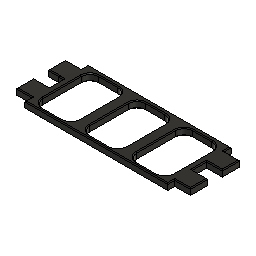
Ansamblu Final (Autodesk Fusion 360 archive; units mm, degrees)
design "Cadran Numere"
part number: 2026-05-27-02-16-51-186
Autodesk Fusion 360 part; units mm, degrees
(part 1 of 3)
sketch "Sketch1" plane through (0, 0, 0) normal (0, 0, 1) x (1, 0, 0)
  line L0 (40, 20) -> (128, 20)
  line L1 (40, 20) -> (40, 24)
  line L2 (40, 24) -> (34, 24)
  line L3 (34, 24) -> (34, 34)
  line L4 (34, 34) -> (40, 34)
  line L5 (40, 34) -> (40, 42.3)
  line L6 (40, 42.3) -> (34, 42.3)
  line L7 (34, 42.3) -> (34, 52.3)
  line L8 (34, 52.3) -> (40, 52.3)
  line L9 (40, 52.3) -> (40, 56.3)
  line L10 (40, 56.3) -> (128, 56.3)
  line L11 (128, 56.3) -> (128, 52.3)
  line L12 (128, 52.3) -> (134, 52.3)
  line L13 (134, 52.3) -> (134, 42.3)
  line L14 (134, 42.3) -> (128, 42.3)
  line L15 (128, 42.3) -> (128, 34)
  line L16 (128, 34) -> (134, 34)
  line L17 (134, 34) -> (134, 24)
  line L18 (134, 24) -> (128, 24)
  line L19 (128, 24) -> (128, 20)
  line L20 (51.5, 53.8) -> (62.5, 53.8)
  line L21 (67.5, 48.8) -> (67.5, 26.8)
  line L22 (62.5, 21.8) -> (51.5, 21.8)
  line L23 (46.5, 26.8) -> (46.5, 48.8)
  line L24 (78.5, 53.8) -> (89.5, 53.8)
  line L25 (94.5, 48.8) -> (94.5, 26.8)
  line L26 (89.5, 21.8) -> (78.5, 21.8)
  line L27 (73.5, 26.8) -> (73.5, 48.8)
  line L28 (105.5, 53.8) -> (116.5, 53.8)
  line L29 (121.5, 48.8) -> (121.5, 26.8)
  line L30 (116.5, 21.8) -> (105.5, 21.8)
  line L31 (100.5, 26.8) -> (100.5, 48.8)
  arc A0 (51.5, 53.8) -> (46.5, 48.8) centre (51.5, 48.8) ccw
  arc A1 (67.5, 48.8) -> (62.5, 53.8) centre (62.5, 48.8) ccw
  arc A2 (46.5, 26.8) -> (51.5, 21.8) centre (51.5, 26.8) ccw
  arc A3 (62.5, 21.8) -> (67.5, 26.8) centre (62.5, 26.8) ccw
  arc A4 (78.5, 53.8) -> (73.5, 48.8) centre (78.5, 48.8) ccw
  arc A5 (73.5, 26.8) -> (78.5, 21.8) centre (78.5, 26.8) ccw
  arc A6 (89.5, 21.8) -> (94.5, 26.8) centre (89.5, 26.8) ccw
  arc A7 (94.5, 48.8) -> (89.5, 53.8) centre (89.5, 48.8) ccw
  arc A8 (105.5, 53.8) -> (100.5, 48.8) centre (105.5, 48.8) ccw
  arc A9 (121.5, 48.8) -> (116.5, 53.8) centre (116.5, 48.8) ccw
  arc A10 (100.5, 26.8) -> (105.5, 21.8) centre (105.5, 26.8) ccw
  arc A11 (116.5, 21.8) -> (121.5, 26.8) centre (116.5, 26.8) ccw
  point P0 (46.5, 53.8)
  point P1 (67.5, 53.8)
  point P2 (46.5, 21.8)
  point P3 (73.5, 53.8)
  point P4 (94.5, 53.8)
  point P5 (73.5, 21.8)
  point P6 (100.5, 53.8)
  point P7 (121.5, 53.8)
  point P8 (100.5, 21.8)
  dimension "d1" = 88
  dimension "d2" = 4
  dimension "d3" = 6
  dimension "d4" = 10
  dimension "d5" = 6
  dimension "d6" = 8.3
  dimension "d7" = 6
  dimension "d8" = 10
  dimension "d9" = 6
  dimension "d10" = 4
  dimension "d11" = 88
  dimension "d12" = 4
  dimension "d13" = 6
  dimension "d14" = 10
  dimension "d15" = 6
  dimension "d16" = 8.3
  dimension "d17" = 6
  dimension "d18" = 10
  dimension "d21" = 21
  dimension "d22" = 32
  dimension "d23" = 6
  dimension "d24" = 21
  dimension "d25" = 32
  dimension "d26" = 6
  dimension "d27" = 21
  dimension "d28" = 32
  dimension "d29" = 5
  constraint horizontal L0
  constraint perpendicular L0 L1
  constraint perpendicular L1 L2
  constraint perpendicular L2 L3
  constraint perpendicular L3 L4
  constraint perpendicular L4 L5
  constraint perpendicular L5 L6
  constraint perpendicular L6 L7
  constraint perpendicular L7 L8
  constraint perpendicular L8 L9
  constraint perpendicular L9 L10
  constraint perpendicular L10 L11
  constraint perpendicular L11 L12
  constraint perpendicular L12 L13
  constraint perpendicular L13 L14
  constraint perpendicular L14 L15
  constraint perpendicular L15 L16
  constraint perpendicular L16 L17
  constraint perpendicular L17 L18
  constraint horizontal L20
  constraint vertical L21
  constraint horizontal L22
  constraint vertical L23
  constraint horizontal L24
  constraint vertical L25
  constraint horizontal L26
  constraint vertical L27
  constraint horizontal L28
  constraint vertical L29
  constraint horizontal L30
  constraint vertical L31
  constraint coincident P0 L20
  constraint coincident P0 L23
  constraint tangent L20 A0
  constraint tangent L23 A0
  constraint coincident P1 L20
  constraint coincident P1 L21
  constraint tangent L20 A1
  constraint tangent L21 A1
  constraint equal A0 A1
  constraint coincident P2 L23
  constraint coincident P2 L22
  constraint tangent L23 A2
  constraint tangent L22 A2
  constraint equal A0 A2
  constraint tangent L21 A3
  constraint tangent L22 A3
  constraint equal A0 A3
  constraint coincident P3 L24
  constraint coincident P3 L27
  constraint tangent L24 A4
  constraint tangent L27 A4
  constraint equal A0 A4
  constraint coincident P5 L27
  constraint coincident P5 L26
  constraint tangent L27 A5
  constraint tangent L26 A5
  constraint equal A0 A5
  constraint tangent L26 A6
  constraint tangent L25 A6
  constraint equal A0 A6
  constraint coincident P4 L25
  constraint coincident P4 L24
  constraint tangent L25 A7
  constraint tangent L24 A7
  constraint equal A0 A7
  constraint coincident P6 L28
  constraint coincident P6 L31
  constraint tangent L28 A8
  constraint tangent L31 A8
  constraint equal A0 A8
  constraint coincident P7 L28
  constraint coincident P7 L29
  constraint tangent L28 A9
  constraint tangent L29 A9
  constraint equal A0 A9
  constraint coincident P8 L31
  constraint coincident P8 L30
  constraint tangent L31 A10
  constraint tangent L30 A10
  constraint equal A0 A10
  constraint tangent L29 A11
  constraint tangent L30 A11
  constraint equal A0 A11
  measures "d1" distance of L0.start L0.end
  measures "d2" distance of L0.start L1.end
  measures "d3" distance of L1.end L2.end
  measures "d4" distance of L2.end L3.end
  measures "d5" distance of L3.end L4.end
  measures "d6" distance of L4.end L5.end
  measures "d7" distance of L5.end L6.end
  measures "d8" distance of L6.end L7.end
  measures "d9" distance of L7.end L8.end
  measures "d10" distance of L8.end L9.end
  measures "d11" distance of L9.end L10.end
  measures "d12" distance of L10.end L11.end
  measures "d13" distance of L11.end L12.end
  measures "d14" distance of L12.end L13.end
  measures "d15" distance of L13.end L14.end
  measures "d16" distance of L14.end L15.end
  measures "d17" distance of L15.end L16.end
  measures "d18" distance of L16.end L17.end
  measures "d21" distance of P0 P1
  measures "d22" distance of P0 P2
  measures "d23" distance of P1 P3
  measures "d24" distance of P3 P4
  measures "d25" distance of P3 P5
  measures "d26" distance of P4 P6
  measures "d27" distance of P6 P7
  measures "d28" distance of P6 P8
  measures "d29" radius of A0
extrude "Extrude1" add sketch "Sketch1" along normal blind 4
sketch "Sketch2" plane through (0, 0, 4) normal (0, 0, 1) x (-1, 0, 0)
  arc A0 (-100.5, -26.8) -> (-105.5, -21.8) centre (-105.5, -26.8) ccw
  line L0 (-100.5, -26.8) -> (-100.5, -48.8)
  arc A1 (-105.5, -53.8) -> (-100.5, -48.8) centre (-105.5, -48.8) ccw
  line L1 (-105.5, -53.8) -> (-116.5, -53.8)
  arc A2 (-121.5, -48.8) -> (-116.5, -53.8) centre (-116.5, -48.8) ccw
  line L2 (-121.5, -48.8) -> (-121.5, -26.8)
  arc A3 (-116.5, -21.8) -> (-121.5, -26.8) centre (-116.5, -26.8) ccw
  line L3 (-116.5, -21.8) -> (-105.5, -21.8)
  arc A4 (-89.5, -21.8) -> (-94.5, -26.8) centre (-89.5, -26.8) ccw
  line L4 (-89.5, -21.8) -> (-78.5, -21.8)
  arc A5 (-73.5, -26.8) -> (-78.5, -21.8) centre (-78.5, -26.8) ccw
  line L5 (-73.5, -26.8) -> (-73.5, -48.8)
  arc A6 (-78.5, -53.8) -> (-73.5, -48.8) centre (-78.5, -48.8) ccw
  line L6 (-78.5, -53.8) -> (-89.5, -53.8)
  arc A7 (-94.5, -48.8) -> (-89.5, -53.8) centre (-89.5, -48.8) ccw
  line L7 (-94.5, -48.8) -> (-94.5, -26.8)
  arc A8 (-46.5, -26.8) -> (-51.5, -21.8) centre (-51.5, -26.8) ccw
  line L8 (-46.5, -26.8) -> (-46.5, -48.8)
  arc A9 (-51.5, -53.8) -> (-46.5, -48.8) centre (-51.5, -48.8) ccw
  line L9 (-51.5, -53.8) -> (-62.5, -53.8)
  arc A10 (-67.5, -48.8) -> (-62.5, -53.8) centre (-62.5, -48.8) ccw
  line L10 (-67.5, -48.8) -> (-67.5, -26.8)
  arc A11 (-62.5, -21.8) -> (-67.5, -26.8) centre (-62.5, -26.8) ccw
  line L11 (-62.5, -21.8) -> (-51.5, -21.8)
  line L12 (-40, -20) -> (-128, -20)
  line L13 (-128, -20) -> (-128, -24)
  line L14 (-128, -24) -> (-134, -24)
  line L15 (-134, -24) -> (-134, -34)
  line L16 (-134, -34) -> (-128, -34)
  line L17 (-128, -34) -> (-128, -42.3)
  line L18 (-128, -42.3) -> (-134, -42.3)
  line L19 (-134, -42.3) -> (-134, -52.3)
  line L20 (-134, -52.3) -> (-128, -52.3)
  line L21 (-128, -52.3) -> (-128, -56.3)
  line L22 (-128, -56.3) -> (-40, -56.3)
  line L23 (-40, -56.3) -> (-40, -52.3)
  line L24 (-40, -52.3) -> (-34, -52.3)
  line L25 (-34, -52.3) -> (-34, -42.3)
  line L26 (-34, -42.3) -> (-40, -42.3)
  line L27 (-40, -42.3) -> (-40, -34)
  line L28 (-40, -34) -> (-34, -34)
  line L29 (-34, -34) -> (-34, -24)
  line L30 (-34, -24) -> (-40, -24)
  line L31 (-40, -24) -> (-40, -20)
  line L32 (-40, -56.3) -> (-43, -56.3)
  line L33 (-43, -56.3) -> (-43, -20)
  line L34 (-43, -20) -> (-40, -20)
  line L35 (-40, -20) -> (-40, -56.3)
  line L36 (-128, -56.3) -> (-125, -56.3)
  line L37 (-125, -56.3) -> (-125, -20)
  line L38 (-125, -20) -> (-128, -20)
  line L39 (-128, -20) -> (-128, -56.3)
  line L40 (-128, -52.3) -> (-125, -52.3)
  line L41 (-125, -52.3) -> (-125, -42.3)
  line L42 (-125, -42.3) -> (-128, -42.3)
  line L43 (-128, -42.3) -> (-128, -52.3)
  line L44 (-128, -34) -> (-125, -34)
  line L45 (-125, -34) -> (-125, -24)
  line L46 (-125, -24) -> (-128, -24)
  line L47 (-128, -24) -> (-128, -34)
  line L48 (-40, -52.3) -> (-43, -52.3)
  line L49 (-43, -52.3) -> (-43, -42)
  line L50 (-43, -42) -> (-40, -42)
  line L51 (-40, -42) -> (-40, -52.3)
  line L52 (-40, -34) -> (-43, -34)
  line L53 (-43, -34) -> (-43, -24)
  line L54 (-43, -24) -> (-40, -24)
  line L55 (-40, -24) -> (-40, -34)
  line L56 (-40, -42) -> (-43, -42)
  line L57 (-43, -42) -> (-43, -34)
  line L58 (-43, -34) -> (-40, -34)
  line L59 (-40, -34) -> (-40, -42)
  line L60 (-40, -56.3) -> (-43, -56.3)
  line L61 (-43, -56.3) -> (-43, -52.3)
  line L62 (-43, -52.3) -> (-40, -52.3)
  line L63 (-40, -52.3) -> (-40, -56.3)
  line L64 (-40, -24) -> (-43, -24)
  line L65 (-43, -24) -> (-43, -20)
  line L66 (-43, -20) -> (-40, -20)
  line L67 (-40, -20) -> (-40, -24)
  line L68 (-125, -56.3) -> (-128, -56.3)
  line L69 (-128, -56.3) -> (-128, -52.3)
  line L70 (-128, -52.3) -> (-125, -52.3)
  line L71 (-125, -52.3) -> (-125, -56.3)
  line L72 (-125, -42.3) -> (-128, -42.3)
  line L73 (-128, -42.3) -> (-128, -34)
  line L74 (-128, -34) -> (-125, -34)
  line L75 (-125, -34) -> (-125, -42.3)
  line L76 (-125, -24) -> (-128, -24)
  line L77 (-128, -24) -> (-128, -20)
  line L78 (-128, -20) -> (-125, -20)
  line L79 (-125, -20) -> (-125, -24)
  constraint horizontal L32
  constraint vertical L33
  constraint horizontal L34
  constraint vertical L35
  constraint coincident L12 L33.end
  constraint coincident L22.end L23.start
  constraint horizontal L36
  constraint vertical L37
  constraint horizontal L38
  constraint vertical L39
  constraint coincident L12 L37.end
  constraint coincident L21.end L22.start
  constraint horizontal L40
  constraint vertical L41
  constraint horizontal L42
  constraint vertical L43
  constraint coincident L37 L41.end
  constraint coincident L20.end L21.start
  constraint horizontal L44
  constraint vertical L45
  constraint horizontal L46
  constraint vertical L47
  constraint coincident L37 L45.end
  constraint coincident L16.end L17.start
  constraint horizontal L48
  constraint vertical L49
  constraint horizontal L50
  constraint vertical L51
  constraint coincident L33 L49.end
  constraint coincident L23.end L24.start
  constraint horizontal L52
  constraint vertical L53
  constraint horizontal L54
  constraint vertical L55
  constraint coincident L33 L53.end
  constraint coincident L27.end L28.start
  constraint horizontal L56
  constraint vertical L57
  constraint horizontal L58
  constraint vertical L59
  constraint horizontal L60
  constraint vertical L61
  constraint horizontal L62
  constraint vertical L63
  constraint horizontal L64
  constraint vertical L65
  constraint horizontal L66
  constraint vertical L67
  constraint horizontal L68
  constraint vertical L69
  constraint horizontal L70
  constraint vertical L71
  constraint horizontal L72
  constraint vertical L73
  constraint horizontal L74
  constraint vertical L75
  constraint horizontal L76
  constraint vertical L77
  constraint horizontal L78
  constraint vertical L79
extrude "Extrude2" cut sketch "Sketch2" against normal blind 40 contours L12 L31 L33 L34 L35 L54 L64 L65 L66 L67 | L12 L13 L37 L38 L39 L46 L76 L77 L78 L79 | L27 L33 L35 L50 L52 L56 L57 L58 L59 | L17 L37 L39 L42 L44 L72 L73 L74 L75 | L22 L23 L32 L33 L35 L48 L60 L61 L62 L63 | L21 L22 L36 L37 L39 L40 L68 L69 L70 L71
chamfer "Chamfer1" distance 0.5 angle 45 1 faces at (39, 30.6667, 4)
chamfer "Chamfer2" distance 0.5 angle 45 1 faces at (39, 30.6667, 0)

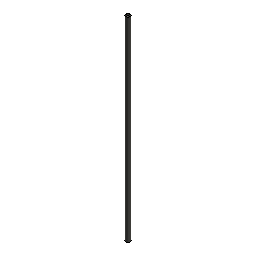
design "Tija"
part number: 2026-05-28-21-26-40-554
Autodesk Fusion 360 part; units mm, degrees
sketch "Sketch1" plane through (0, 0, 0) normal (0, 0, 1) x (1, 0, 0)
  circle A0 centre (8.6658, 10.0855) radius 1.15
  dimension "d1" = 2.3
  measures "d1" diameter of A0
extrude "Extrude1" add sketch "Sketch1" along normal blind 120
extrude "Extrude2" cut 1 faces at (8.9089, 10.1799, 120) along direction (0, 0, -1) blind 20
chamfer "Chamfer1" distance 0.5 angle 45 2 faces at (8.9089, 10.1799, 100) (9.7701, 9.7644, 33.3333)

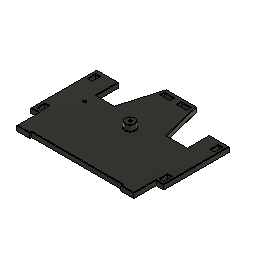
design "Rama stanga"
part number: 2026-05-28-04-13-53-551
Autodesk Fusion 360 part; units mm, degrees
sketch "Sketch1" plane through (0, 0, 0) normal (0, 0, 1) x (1, 0, 0)
  line L0 (27.8497, 75.8381) -> (51.8497, 75.8381)
  line L1 (51.8497, 75.8381) -> (51.8497, 51.1381)
  line L2 (51.8497, 51.1381) -> (71.8497, 51.1381)
  line L3 (71.8497, 51.1381) -> (84.8497, 95.4381)
  line L4 (84.8497, 95.4381) -> (117.8497, 95.4381)
  line L5 (117.8497, 95.4381) -> (128.8497, 51.4381)
  line L6 (128.8497, 51.4381) -> (151.8497, 51.4381)
  line L7 (151.8497, 51.4381) -> (151.8497, 75.4381)
  line L8 (151.8497, 75.4381) -> (173.8497, 75.4381)
  line L9 (173.8497, 75.4381) -> (173.8497, 3.4381)
  line L10 (173.8497, 3.4381) -> (165.4497, 3.4381)
  line L11 (165.4497, 3.4381) -> (165.4497, -21.0619)
  line L12 (165.4497, -21.0619) -> (151.0497, -21.0619)
  line L13 (151.0497, -21.0619) -> (151.0497, -19.0619)
  line L14 (151.0497, -19.0619) -> (51.0497, -19.0619)
  line L15 (51.0497, -19.0619) -> (51.0497, -21.0619)
  line L16 (51.0497, -21.0619) -> (36.7497, -21.0619)
  line L17 (36.7497, -21.0619) -> (36.7497, 3.4381)
  line L18 (36.7497, 3.4381) -> (27.7497, 3.4381)
  line L19 (27.7497, 3.4381) -> (27.8497, 75.8381)
  line L20 (31.5497, 71.033) -> (35.8497, 71.033)
  line L21 (35.8497, 71.033) -> (35.8497, 62.733)
  line L22 (35.8497, 62.733) -> (31.5497, 62.733)
  line L23 (31.5497, 62.733) -> (31.5497, 71.033)
  line L24 (31.4497, 6.933) -> (35.7497, 6.933)
  line L25 (35.7497, 6.933) -> (35.7497, 15.233)
  line L26 (35.7497, 15.233) -> (31.4497, 15.233)
  line L27 (31.4497, 15.233) -> (31.4497, 6.933)
  line L28 (170.5497, 70.9381) -> (166.2497, 70.9381)
  line L29 (166.2497, 70.9381) -> (166.2497, 62.6381)
  line L30 (166.2497, 62.6381) -> (170.5497, 62.6381)
  line L31 (170.5497, 62.6381) -> (170.5497, 70.9381)
  line L32 (170.5497, 6.9381) -> (166.2497, 6.9381)
  line L33 (166.2497, 6.9381) -> (166.2497, 15.2381)
  line L34 (166.2497, 15.2381) -> (170.5497, 15.2381)
  line L35 (170.5497, 15.2381) -> (170.5497, 6.9381)
  line L36 (86.7497, 91.2381) -> (97.0497, 91.2381)
  line L37 (97.0497, 91.2381) -> (97.0497, 86.9381)
  line L38 (97.0497, 86.9381) -> (86.7497, 86.9381)
  line L39 (86.7497, 86.9381) -> (86.7497, 91.2381)
  line L40 (105.0497, 91.2381) -> (115.3497, 91.2381)
  line L41 (115.3497, 91.2381) -> (115.3497, 86.9381)
  line L42 (115.3497, 86.9381) -> (105.0497, 86.9381)
  line L43 (105.0497, 86.9381) -> (105.0497, 91.2381)
  line L44 (84.8497, 95.4381) -> (101.3497, 95.4381)
  circle A0 centre (101.3497, 38.9381) radius 1.25
  circle A1 centre (101.3497, 38.9381) radius 5.5
  circle A2 centre (51.3497, 38.9381) radius 1.25
  dimension "d1" = 24
  dimension "d2" = 24.7
  dimension "d3" = 20
  dimension "d6" = 33
  dimension "d9" = 23
  dimension "d10" = 24
  dimension "d11" = 22
  dimension "d12" = 72
  dimension "d13" = 8.4
  dimension "d14" = 24.5
  dimension "d15" = 14.4
  dimension "d16" = 2
  dimension "d17" = 100
  dimension "d18" = 2
  dimension "d19" = 14.3
  dimension "d20" = 24.5
  dimension "d21" = 9
  dimension "d24" = 4.3
  dimension "d25" = 8.3
  dimension "d28" = 4.3
  dimension "d29" = 8.3
  dimension "d32" = 4.3
  dimension "d33" = 8.3
  dimension "d36" = 4.3
  dimension "d37" = 8.3
  dimension "d40" = 10.3
  dimension "d41" = 4.3
  dimension "d42" = 8
  dimension "d43" = 10.3
  dimension "d44" = 4.3
  dimension "d45" = 56.5
  dimension "d46" = 2.5
  dimension "d47" = 11
  dimension "d48" = 50
  dimension "d49" = 2.5
  constraint horizontal L0
  constraint perpendicular L0 L1
  constraint perpendicular L1 L2
  constraint perpendicular L6 L7
  constraint perpendicular L7 L8
  constraint perpendicular L8 L9
  constraint perpendicular L9 L10
  constraint perpendicular L10 L11
  constraint perpendicular L11 L12
  constraint vertical L13
  constraint perpendicular L13 L14
  constraint perpendicular L14 L15
  constraint perpendicular L15 L16
  constraint perpendicular L16 L17
  constraint perpendicular L17 L18
  constraint horizontal L20
  constraint vertical L21
  constraint horizontal L22
  constraint vertical L23
  constraint horizontal L24
  constraint vertical L25
  constraint horizontal L26
  constraint vertical L27
  constraint horizontal L28
  constraint vertical L29
  constraint horizontal L30
  constraint vertical L31
  constraint horizontal L32
  constraint vertical L33
  constraint horizontal L34
  constraint vertical L35
  constraint horizontal L36
  constraint vertical L37
  constraint horizontal L38
  constraint vertical L39
  constraint horizontal L40
  constraint vertical L41
  constraint horizontal L42
  constraint vertical L43
  constraint midpoint L4 L44.end
  constraint concentric A0 A1
  measures "d1" distance of L0.start L0.end
  measures "d2" distance of L0.end L1.end
  measures "d3" distance of L1.end L2.end
  measures "d6" distance of L3.end L4.end
  measures "d9" distance of L5.end L6.end
  measures "d10" distance of L6.end L7.end
  measures "d11" distance of L7.end L8.end
  measures "d12" distance of L8.end L9.end
  measures "d13" distance of L9.end L10.end
  measures "d14" distance of L10.end L11.end
  measures "d15" distance of L11.end L12.end
  measures "d16" distance of L12.end L13.end
  measures "d17" distance of L13.end L14.end
  measures "d18" distance of L14.end L15.end
  measures "d19" distance of L15.end L16.end
  measures "d20" distance of L16.end L17.end
  measures "d21" distance of L17.end L18.end
  measures "d24" distance of L20.start L20.end
  measures "d25" distance of L20.start L22.end
  measures "d28" distance of L24.start L24.end
  measures "d29" distance of L24.start L26.end
  measures "d32" distance of L28.start L28.end
  measures "d33" distance of L28.start L30.end
  measures "d36" distance of L32.start L32.end
  measures "d37" distance of L32.start L34.end
  measures "d40" distance of L36.start L36.end
  measures "d41" distance of L36.start L38.end
  measures "d42" distance of L36.end L40.start
  measures "d43" distance of L40.start L40.end
  measures "d44" distance of L40.start L42.end
  measures "d45" distance of L44.end A0.centre
  measures "d46" diameter of A0
  measures "d47" diameter of A1
  measures "d48" distance of A0.centre A2.centre
  measures "d49" diameter of A2
extrude "Extrude1" add sketch "Sketch1" along normal blind 6 contours L0 L1 L2 L3 L4 L5 L6 L7 L8 L9 L10 L11 L12 L13 L14 L15 L16 L17 L18 L19 L44
extrude "Extrude2" add sketch "Sketch1" along normal blind 12.5 contours A1
chamfer "Chamfer1" distance 0.5 angle 45 1 faces at (101.0127, -1.5568, 6)
chamfer "Chamfer2" distance 0.3 angle 45 1 faces at (105.4126, 38.6648, 12.5)
chamfer "Chamfer3" distance 0.5 angle 45 1 faces at (101.0904, -0.141, 0)

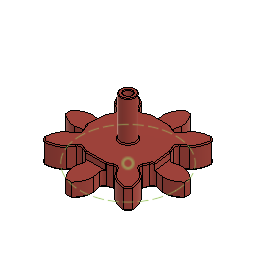
design "Roata mica"
part number: 2026-05-27-03-58-10-085
description: Spur Gear; Module: 3.6; Num Teeth: 8; Pressure Angle: 20.0; Backlash: 0.00 mm
part number: 2026-05-27-04-00-53-761
part number: 2026-05-27-04-03-58-853
Autodesk Fusion 360 part; units mm, degrees
sketch "Base Circle" plane through (0, 0, 0) normal (0, 0, 1) x (1, 0, 0) in component "Spur Gear 8 teeth"
  circle A0 centre (0, 0) radius 10.2348
  circle A1 centre (0, 0) radius 1.15
extrude "Extrude1" add sketch "Base Circle" along normal blind 4.5 contours A0 picked at (7.168429, -0.508473) makes body 1 in component "Spur Gear 8 teeth"
sketch "Gear Tooth" plane through (0, 0, 0) normal (0, 0, 1) x (1, 0, 0) in component "Spur Gear 8 teeth"
  spline S0 degree 5 poles (13.23075, -2.837383) (13.244003, -2.840225) (13.270575, -2.8454) (13.310634, -2.851636) (13.364425, -2.857051) (13.432189, -2.859891) (13.500337, -2.859938) (13.56873, -2.858297) (13.637265, -2.855743) (13.705893, -2.852533) (13.774606, -2.848599) (13.843415, -2.843687) (13.912339, -2.837503) (13.981384, -2.829877) (14.05054, -2.820834) (14.119787, -2.810501) (14.189099, -2.799061) (14.258453, -2.786693) (14.327831, -2.773501) (14.397224, -2.75951) (14.46663, -2.744699) (14.536047, -2.729023) (14.605473, -2.712438) (14.674904, -2.694933) (14.744334, -2.676527) (14.813755, -2.657255) (14.883156, -2.637157) (14.952531, -2.616273) (15.021871, -2.594626) (15.091173, -2.572224) (15.160431, -2.54907) (15.229641, -2.525161) (15.298799, -2.500496) (15.367901, -2.475081) (15.436941, -2.448924) (15.505915, -2.422038) (15.574817, -2.394436) (15.643643, -2.36613) (15.712387, -2.337129) (15.781046, -2.30744) (15.849615, -2.277067) (15.91809, -2.246015) (15.986467, -2.214289) (16.054742, -2.181892) (16.122912, -2.148832) (16.190971, -2.115115) (16.258916, -2.080748) (16.326743, -2.045735) (16.394449, -2.010083) (16.462029, -1.973797) (16.529479, -1.936882) (16.596797, -1.899341) (16.663979, -1.861179) (16.73102, -1.8224) (16.797918, -1.783009) (16.864669, -1.743011) (16.931268, -1.70241) (16.997713, -1.661209) (17.064, -1.619414) (17.130127, -1.577028) (17.196091, -1.534055) (17.261887, -1.490498) (17.327515, -1.446361) (17.392968, -1.401648) (17.458244, -1.356364) (17.523339, -1.310511) (17.588249, -1.264095) (17.652969, -1.217118) (17.717499, -1.169585) (17.781836, -1.121497) (17.845981, -1.072858) (17.897141, -1.033505) (17.935424, -1.003743) (17.960908, -0.983792) (17.97364, -0.973788) knots 0 0 0 0 0 0 0.01428571 0.02857143 0.04285714 0.05714286 0.07142857 0.08571429 0.1 0.11428571 0.12857143 0.14285714 0.15714286 0.17142857 0.18571429 0.2 0.21428571 0.22857143 0.24285714 0.25714286 0.27142857 0.28571429 0.3 0.31428571 0.32857143 0.34285714 0.35714286 0.37142857 0.38571429 0.4 0.41428571 0.42857143 0.44285714 0.45714286 0.47142857 0.48571429 0.5 0.51428571 0.52857143 0.54285714 0.55714286 0.57142857 0.58571429 0.6 0.61428571 0.62857143 0.64285714 0.65714286 0.67142857 0.68571429 0.7 0.71428571 0.72857143 0.74285714 0.75714286 0.77142857 0.78571429 0.8 0.81428571 0.82857143 0.84285714 0.85714286 0.87142857 0.88571429 0.9 0.91428571 0.92857143 0.94285714 0.95714286 0.97142857 0.98571429 1 1 1 1 1 1
  spline S1 degree 5 poles (13.23075, 2.837383) (13.244003, 2.840225) (13.270575, 2.8454) (13.310634, 2.851636) (13.364425, 2.857051) (13.432189, 2.859891) (13.500337, 2.859938) (13.56873, 2.858297) (13.637265, 2.855743) (13.705893, 2.852533) (13.774606, 2.848599) (13.843415, 2.843687) (13.912339, 2.837503) (13.981384, 2.829877) (14.05054, 2.820834) (14.119787, 2.810501) (14.189099, 2.799061) (14.258453, 2.786693) (14.327831, 2.773501) (14.397224, 2.75951) (14.46663, 2.744699) (14.536047, 2.729023) (14.605473, 2.712438) (14.674904, 2.694933) (14.744334, 2.676527) (14.813755, 2.657255) (14.883156, 2.637157) (14.952531, 2.616273) (15.021871, 2.594626) (15.091173, 2.572224) (15.160431, 2.54907) (15.229641, 2.525161) (15.298799, 2.500496) (15.367901, 2.475081) (15.436941, 2.448924) (15.505915, 2.422038) (15.574817, 2.394436) (15.643643, 2.36613) (15.712387, 2.337129) (15.781046, 2.30744) (15.849615, 2.277067) (15.91809, 2.246015) (15.986467, 2.214289) (16.054742, 2.181892) (16.122912, 2.148832) (16.190971, 2.115115) (16.258916, 2.080748) (16.326743, 2.045735) (16.394449, 2.010083) (16.462029, 1.973797) (16.529479, 1.936882) (16.596797, 1.899341) (16.663979, 1.861179) (16.73102, 1.8224) (16.797918, 1.783009) (16.864669, 1.743011) (16.931268, 1.70241) (16.997713, 1.661209) (17.064, 1.619414) (17.130127, 1.577028) (17.196091, 1.534055) (17.261887, 1.490498) (17.327515, 1.446361) (17.392968, 1.401648) (17.458244, 1.356364) (17.523339, 1.310511) (17.588249, 1.264095) (17.652969, 1.217118) (17.717499, 1.169585) (17.781836, 1.121497) (17.845981, 1.072858) (17.897141, 1.033505) (17.935424, 1.003743) (17.960908, 0.983792) (17.97364, 0.973788) knots 0 0 0 0 0 0 0.01428571 0.02857143 0.04285714 0.05714286 0.07142857 0.08571429 0.1 0.11428571 0.12857143 0.14285714 0.15714286 0.17142857 0.18571429 0.2 0.21428571 0.22857143 0.24285714 0.25714286 0.27142857 0.28571429 0.3 0.31428571 0.32857143 0.34285714 0.35714286 0.37142857 0.38571429 0.4 0.41428571 0.42857143 0.44285714 0.45714286 0.47142857 0.48571429 0.5 0.51428571 0.52857143 0.54285714 0.55714286 0.57142857 0.58571429 0.6 0.61428571 0.62857143 0.64285714 0.65714286 0.67142857 0.68571429 0.7 0.71428571 0.72857143 0.74285714 0.75714286 0.77142857 0.78571429 0.8 0.81428571 0.82857143 0.84285714 0.85714286 0.87142857 0.88571429 0.9 0.91428571 0.92857143 0.94285714 0.95714286 0.97142857 0.98571429 1 1 1 1 1 1
  arc A0 (17.97364, -0.973788) -> (17.97364, 0.973788) centre (0, 0) ccw
  line L0 (9.99749, -2.143999) -> (13.23075, -2.837383)
  line L1 (9.99749, 2.143999) -> (13.23075, 2.837383)
  line L2 (9.99749, -2.143999) -> (9.99749, 2.143999)
  point P0 (13.552566, -2.858522)
  point P1 (13.882397, -2.840016)
  point P2 (14.217163, -2.793942)
  point P3 (14.555525, -2.724234)
  point P4 (14.896536, -2.632993)
  point P5 (15.239415, -2.521529)
  point P6 (15.583466, -2.390735)
  point P7 (15.928048, -2.24126)
  point P8 (16.272548, -2.073591)
  point P9 (16.616378, -1.888116)
  point P10 (16.958962, -1.685148)
  point P11 (17.299738, -1.464954)
  point P12 (17.638147, -1.227764)
  point P13 (13.552566, 2.858522)
  point P14 (13.882397, 2.840016)
  point P15 (14.217163, 2.793942)
  point P16 (14.555525, 2.724234)
  point P17 (14.896536, 2.632993)
  point P18 (15.239415, 2.521529)
  point P19 (15.583466, 2.390735)
  point P20 (15.928048, 2.24126)
  point P21 (16.272548, 2.073591)
  point P22 (16.616378, 1.888116)
  point P23 (16.958962, 1.685148)
  point P24 (17.299738, 1.464954)
  point P25 (17.638147, 1.227764)
extrude "Extrude2" add sketch "Gear Tooth" along normal blind 4.5 contours S0 S1 A0 L0 L1 L2 picked at (12.152997, -0.714666) bodies 1 in component "Spur Gear 8 teeth"
fillet "Fillet1" radius 1.2 2 edges at (10.007268, -2.146095, 2.25) (10.007268, 2.146095, 2.25) on bodies 1 in component "Spur Gear 8 teeth"
pattern_circular "C-Pattern1" count 8 over 360 about axis through (0, 0, 0) along (0, 0, 1) of "Extrude2", "Fillet1" in component "Spur Gear 8 teeth"
sketch "Diametrial Pitch Circle" plane through (0, 0, 0) normal (0, 0, 1) x (1, 0, 0) in component "Spur Gear 8 teeth"
  circle A0 centre (0, 0) radius 14.4 construction
sketch "Base Circle (2)" plane through (0, 0, 0) normal (0, 0, 1) x (1, 0, 0) in component "Spur Gear 8 teeth (1)"
  circle A0 centre (0, 0) radius 10.2348
  circle A1 centre (0, 0) radius 1.15
extrude "Extrude1'" add sketch "Base Circle (2)" along normal blind 6.5 separate body contours A0 picked at (7.168429, -0.508473) makes body 2 in component "Spur Gear 8 teeth (1)"
sketch "Gear Tooth (2)" plane through (0, 0, 0) normal (0, 0, 1) x (1, 0, 0) in component "Spur Gear 8 teeth (1)"
  spline S0 degree 5 poles (13.23075, -2.837383) (13.244003, -2.840225) (13.270575, -2.8454) (13.310634, -2.851636) (13.364425, -2.857051) (13.432189, -2.859891) (13.500337, -2.859938) (13.56873, -2.858297) (13.637265, -2.855743) (13.705893, -2.852533) (13.774606, -2.848599) (13.843415, -2.843687) (13.912339, -2.837503) (13.981384, -2.829877) (14.05054, -2.820834) (14.119787, -2.810501) (14.189099, -2.799061) (14.258453, -2.786693) (14.327831, -2.773501) (14.397224, -2.75951) (14.46663, -2.744699) (14.536047, -2.729023) (14.605473, -2.712438) (14.674904, -2.694933) (14.744334, -2.676527) (14.813755, -2.657255) (14.883156, -2.637157) (14.952531, -2.616273) (15.021871, -2.594626) (15.091173, -2.572224) (15.160431, -2.54907) (15.229641, -2.525161) (15.298799, -2.500496) (15.367901, -2.475081) (15.436941, -2.448924) (15.505915, -2.422038) (15.574817, -2.394436) (15.643643, -2.36613) (15.712387, -2.337129) (15.781046, -2.30744) (15.849615, -2.277067) (15.91809, -2.246015) (15.986467, -2.214289) (16.054742, -2.181892) (16.122912, -2.148832) (16.190971, -2.115115) (16.258916, -2.080748) (16.326743, -2.045735) (16.394449, -2.010083) (16.462029, -1.973797) (16.529479, -1.936882) (16.596797, -1.899341) (16.663979, -1.861179) (16.73102, -1.8224) (16.797918, -1.783009) (16.864669, -1.743011) (16.931268, -1.70241) (16.997713, -1.661209) (17.064, -1.619414) (17.130127, -1.577028) (17.196091, -1.534055) (17.261887, -1.490498) (17.327515, -1.446361) (17.392968, -1.401648) (17.458244, -1.356364) (17.523339, -1.310511) (17.588249, -1.264095) (17.652969, -1.217118) (17.717499, -1.169585) (17.781836, -1.121497) (17.845981, -1.072858) (17.897141, -1.033505) (17.935424, -1.003743) (17.960908, -0.983792) (17.97364, -0.973788) knots 0 0 0 0 0 0 0.01428571 0.02857143 0.04285714 0.05714286 0.07142857 0.08571429 0.1 0.11428571 0.12857143 0.14285714 0.15714286 0.17142857 0.18571429 0.2 0.21428571 0.22857143 0.24285714 0.25714286 0.27142857 0.28571429 0.3 0.31428571 0.32857143 0.34285714 0.35714286 0.37142857 0.38571429 0.4 0.41428571 0.42857143 0.44285714 0.45714286 0.47142857 0.48571429 0.5 0.51428571 0.52857143 0.54285714 0.55714286 0.57142857 0.58571429 0.6 0.61428571 0.62857143 0.64285714 0.65714286 0.67142857 0.68571429 0.7 0.71428571 0.72857143 0.74285714 0.75714286 0.77142857 0.78571429 0.8 0.81428571 0.82857143 0.84285714 0.85714286 0.87142857 0.88571429 0.9 0.91428571 0.92857143 0.94285714 0.95714286 0.97142857 0.98571429 1 1 1 1 1 1
  spline S1 degree 5 poles (13.23075, 2.837383) (13.244003, 2.840225) (13.270575, 2.8454) (13.310634, 2.851636) (13.364425, 2.857051) (13.432189, 2.859891) (13.500337, 2.859938) (13.56873, 2.858297) (13.637265, 2.855743) (13.705893, 2.852533) (13.774606, 2.848599) (13.843415, 2.843687) (13.912339, 2.837503) (13.981384, 2.829877) (14.05054, 2.820834) (14.119787, 2.810501) (14.189099, 2.799061) (14.258453, 2.786693) (14.327831, 2.773501) (14.397224, 2.75951) (14.46663, 2.744699) (14.536047, 2.729023) (14.605473, 2.712438) (14.674904, 2.694933) (14.744334, 2.676527) (14.813755, 2.657255) (14.883156, 2.637157) (14.952531, 2.616273) (15.021871, 2.594626) (15.091173, 2.572224) (15.160431, 2.54907) (15.229641, 2.525161) (15.298799, 2.500496) (15.367901, 2.475081) (15.436941, 2.448924) (15.505915, 2.422038) (15.574817, 2.394436) (15.643643, 2.36613) (15.712387, 2.337129) (15.781046, 2.30744) (15.849615, 2.277067) (15.91809, 2.246015) (15.986467, 2.214289) (16.054742, 2.181892) (16.122912, 2.148832) (16.190971, 2.115115) (16.258916, 2.080748) (16.326743, 2.045735) (16.394449, 2.010083) (16.462029, 1.973797) (16.529479, 1.936882) (16.596797, 1.899341) (16.663979, 1.861179) (16.73102, 1.8224) (16.797918, 1.783009) (16.864669, 1.743011) (16.931268, 1.70241) (16.997713, 1.661209) (17.064, 1.619414) (17.130127, 1.577028) (17.196091, 1.534055) (17.261887, 1.490498) (17.327515, 1.446361) (17.392968, 1.401648) (17.458244, 1.356364) (17.523339, 1.310511) (17.588249, 1.264095) (17.652969, 1.217118) (17.717499, 1.169585) (17.781836, 1.121497) (17.845981, 1.072858) (17.897141, 1.033505) (17.935424, 1.003743) (17.960908, 0.983792) (17.97364, 0.973788) knots 0 0 0 0 0 0 0.01428571 0.02857143 0.04285714 0.05714286 0.07142857 0.08571429 0.1 0.11428571 0.12857143 0.14285714 0.15714286 0.17142857 0.18571429 0.2 0.21428571 0.22857143 0.24285714 0.25714286 0.27142857 0.28571429 0.3 0.31428571 0.32857143 0.34285714 0.35714286 0.37142857 0.38571429 0.4 0.41428571 0.42857143 0.44285714 0.45714286 0.47142857 0.48571429 0.5 0.51428571 0.52857143 0.54285714 0.55714286 0.57142857 0.58571429 0.6 0.61428571 0.62857143 0.64285714 0.65714286 0.67142857 0.68571429 0.7 0.71428571 0.72857143 0.74285714 0.75714286 0.77142857 0.78571429 0.8 0.81428571 0.82857143 0.84285714 0.85714286 0.87142857 0.88571429 0.9 0.91428571 0.92857143 0.94285714 0.95714286 0.97142857 0.98571429 1 1 1 1 1 1
  arc A0 (17.97364, -0.973788) -> (17.97364, 0.973788) centre (0, 0) ccw
  line L0 (9.99749, -2.143999) -> (13.23075, -2.837383)
  line L1 (9.99749, 2.143999) -> (13.23075, 2.837383)
  line L2 (9.99749, -2.143999) -> (9.99749, 2.143999)
  point P0 (13.552566, -2.858522)
  point P1 (13.882397, -2.840016)
  point P2 (14.217163, -2.793942)
  point P3 (14.555525, -2.724234)
  point P4 (14.896536, -2.632993)
  point P5 (15.239415, -2.521529)
  point P6 (15.583466, -2.390735)
  point P7 (15.928048, -2.24126)
  point P8 (16.272548, -2.073591)
  point P9 (16.616378, -1.888116)
  point P10 (16.958962, -1.685148)
  point P11 (17.299738, -1.464954)
  point P12 (17.638147, -1.227764)
  point P13 (13.552566, 2.858522)
  point P14 (13.882397, 2.840016)
  point P15 (14.217163, 2.793942)
  point P16 (14.555525, 2.724234)
  point P17 (14.896536, 2.632993)
  point P18 (15.239415, 2.521529)
  point P19 (15.583466, 2.390735)
  point P20 (15.928048, 2.24126)
  point P21 (16.272548, 2.073591)
  point P22 (16.616378, 1.888116)
  point P23 (16.958962, 1.685148)
  point P24 (17.299738, 1.464954)
  point P25 (17.638147, 1.227764)
extrude "Extrude2'" add sketch "Gear Tooth (2)" along normal blind 6.5 contours S0 S1 A0 L0 L1 L2 picked at (12.152997, -0.714666) bodies 2 in component "Spur Gear 8 teeth (1)"
fillet "Fillet1'" radius 1.2 2 edges at (10.007268, -2.146095, 3.25) (10.007268, 2.146095, 3.25) on bodies 2 in component "Spur Gear 8 teeth (1)"
pattern_circular "C-Pattern1'" count 8 over 360 about axis through (0, 0, 0) along (0, 0, 1) of "Extrude2'", "Fillet1'" in component "Spur Gear 8 teeth (1)"
sketch "Diametrial Pitch Circle (2)" plane through (0, 0, 0) normal (0, 0, 1) x (1, 0, 0) in component "Spur Gear 8 teeth (1)"
  circle A0 centre (0, 0) radius 14.4 construction